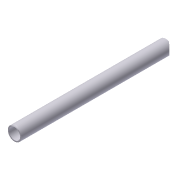
# Autodesk Inventor part: FE-00005-03
Saved by Autodesk Inventor 2012 (Build 160160000, 160)
## iProperties
Company: FIRST
Created: 2008-05-25
Part Number: FE-00005-03
Document SubType Name: Modeling
Designer: dfoster
Density: 1 g/cm^3
Description: Vertical Support
Mass: 200.111 g
Surface Area: 1130.47 cm^2
Volume: 200.111 cm^3
Material: Default
Title: Vertical Support
Author: dfoster
Autodesk Inventor part; units mm, degrees
ref_plane "XZ Plane" through (0, 0, 0) normal (0, 1, 0) x (-1, 0, 0)
ref_plane "XY Plane" through (0, 0, 0) normal (0, 0, 1) x (1, 0, 0)
sketch "Sketch1" plane through (0, 0, 0) normal (0, 0, 1) x (1, 0, 0)
  circle A0 centre (0, 0) radius 21.0312
  circle A1 centre (0, 0) radius 17.4625
  dimension "d0" = 42.0624
  dimension "d1" = 34.925
  constraints: 2 centre point, 1 coincident
  measures "d0" diameter of A0
  measures "d1" diameter of A1
extrude "Extrusion1" add sketch "Sketch1" along normal blind 469.1126
ref_plane "Work Plane1" through (0, 0, 0) normal (1, 0, 0) x (0, 0, 1)
sketch "Sketch2" plane through (0, 0, 0) normal (1, 0, 0) x (0, 0, 1)
  line L0 (0, -21.0312) -> (469.1126, -21.0312) projected
  line L1 (0, -17.4625) -> (0, 17.4625) projected
  line L2 (0, 21.0312) -> (0, -21.0312) projected
  line L3 (-132.8674, 0) -> (569.4426, 0) projected
  line L4 (469.1126, 17.4625) -> (469.1126, -17.4625) projected
  line L5 (469.1126, 21.0312) -> (469.1126, -21.0312) projected
  circle A0 centre (-11.1061, 0) radius 21.4312
  dimension "d5" = 480.2188
  dimension "d6" = 42.8625
  constraints: 1 centre point, 1 point on line
  measures "d5" horizontal distance of L4.end A0.centre
  measures "d6" diameter of A0
extrude "Extrusion2" cut sketch "Sketch2" against normal mid plane 301.625 contours A0 L3 L1 L2 | L2 L1 L3 A0 | A0 L2 L1 L3 | L3 L1 L2 A0
sketch "Sketch3" plane through (0, 0, 0) normal (1, 0, 0) x (0, 0, 1)
  line L0 (0, -21.0312) -> (469.1126, -21.0312) projected
  line L1 (469.1126, 17.4625) -> (469.1126, -17.4625) projected
  line L2 (469.1126, 21.0312) -> (469.1126, -21.0312) projected
  line L3 (443.4545, -21.0312) -> (462.7626, -21.0312)
  line L4 (469.1126, -14.6812) -> (469.1126, -1.9812)
  line L5 (469.1126, -1.9812) -> (508, -1.9812)
  line L6 (508, -1.9812) -> (508, -30.5562)
  line L7 (508, -30.5562) -> (443.4545, -30.5562)
  line L8 (443.4545, -30.5562) -> (443.4545, -21.0312)
  arc A0 (462.7626, -21.0312) -> (469.1126, -14.6812) centre (462.7626, -14.6812) ccw
  dimension "d9" = 6.35
  constraints: 12 end point, 4 parallel, 2 collinear, 2 perpendicular, 2 point on circle, 2 tangent, 1 centre point
  measures "d9" radius of A0
extrude "Extrusion3" cut sketch "Sketch3" against normal mid plane 301.625
body "Solid1"
